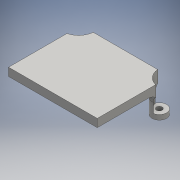
# Autodesk Inventor part: Fan bracket
Saved by Autodesk Inventor 2016 (Build 200138000, 138)
## iProperties
Created: 2019-09-20
Part Number: Fan bracket
Material: Generic
Document SubType Name: Modeling
Designer: jimmy
Density: 1 g/cm^3
Appearance: Default
Author: jimmy
Autodesk Inventor part; units mm, degrees
ref_plane "YZ Plane" through (0, 0, 0) normal (1, 0, 0) x (0, 1, 0)
ref_plane "XZ Plane" through (0, 0, 0) normal (0, 1, 0) x (-1, 0, 0)
ref_plane "XY Plane" through (0, 0, 0) normal (0, 0, 1) x (1, 0, 0)
sketch "Sketch1" plane through (0, 0, 0) normal (0, 0, 1) x (1, 0, 0)
  line L0 (-27.5, 22.5) -> (27.5, 22.5)
  line L1 (27.5, 22.5) -> (27.5, -22.5)
  line L2 (27.5, -22.5) -> (-27.5, -22.5)
  line L3 (-27.5, -22.5) -> (-27.5, 22.5)
  line L4 (-27.5, 22.5) -> (27.5, -22.5) construction
  line L5 (27.5, 22.5) -> (-27.5, -22.5) construction
  point P0 (0, 0)
  dimension "d0" = 55
  dimension "d1" = 45
  constraints: 12 end point, 2 midpoint, 2 parallel, 1 horizontal, 1 perpendicular
  measures "d0" distance of L1.end L2.end
  measures "d1" distance of L0.end L1.end
extrude "Extrusion1" add sketch "Sketch1" along normal blind 5
sketch "Sketch2" plane through (0, 0, 5) normal (0, 0, 1) x (1, 0, 0)
  line L0 (27.5, 22.5) -> (-27.5, 22.5) projected
  line L1 (-27.5, 22.5) -> (-27.5, -22.5) projected
  line L2 (-27.5, -22.5) -> (27.5, -22.5) projected
  line L3 (27.5, -22.5) -> (27.5, 22.5) projected
  line L4 (27.5, 22.5) -> (-27.5, 22.5) projected
  line L5 (27.5, -22.5) -> (27.5, 22.5) projected
  line L6 (-27.5, 22.5) -> (-27.5, -22.5) projected
  circle A0 centre (-24.5, 19) radius 4.5
  circle A1 centre (24.5, 19) radius 4.5
  line L7 (-40.6, 0) -> (40.6, 0) construction
  line L8 (0, -31.5) -> (0, 31.5) construction
  line L9 (-24.5, 19) -> (24.5, 19)
  point P0 (0, 0)
  point P1 (0, 19)
  dimension "d19" = 9
  dimension "d20" = 9
  dimension "d30" = 49
  dimension "d31" = 3.5
  constraints: 2 centre point, 2 end point, 1 horizontal, 1 midpoint, 1 point on line
  measures "d19" diameter of A0
  measures "d20" diameter of A1
  measures "d30" distance of L9.start L9.end
  measures "d31" distance between parallel lines of L9 L0
extrude "Extrusion2" add sketch "Sketch2" against normal blind 20 contours A1 L3 L0 | L0 A1 | A1 L3 | A0 L1 L0 | L0 A0 | L1 A0 picked at (23.9815, 19.6233) picked at (-23.4271, 18.4067)
sketch "Sketch3" plane through (0, 0, 5) normal (0, 0, 1) x (1, 0, 0)
  line L0 (-27.5, 22.5) -> (-27.3284, 22.5) projected
  line L1 (27.5, 22.5) -> (27.5, 22.3541) projected
  line L2 (27.5, -22.5) -> (-27.5, -22.5) projected
  line L3 (-27.5, -22.5) -> (-27.5, 15.6459) projected
  circle A0 centre (-24.5, 19) radius 3
  line L4 (-16.6703, 13.7531) -> (-27.5, 13.7531) construction
  line L5 (-20, 11.9289) -> (-20, 22.5) construction
  arc A1 (-27.5, 13.7531) -> (-20, 22.5) centre (-29.7996, 23.3138) ccw
  line L6 (21.6716, 22.5) -> (-21.6716, 22.5) projected
  line L7 (-27.5, 15.6459) -> (-27.5, -22.5) projected
  arc A2 (21.6716, 22.5) -> (27.5, 15.6459) centre (24.5, 19) ccw projected
  arc A3 (-27.5, 15.6459) -> (-21.6716, 22.5) centre (-24.5, 19) ccw projected
  line L8 (-20, 22.5) -> (-20, 25.8923)
  line L9 (-20, 25.8923) -> (-33.1535, 25.8923)
  line L10 (-33.1535, 25.8923) -> (-33.1535, 13.7531)
  line L11 (-33.1535, 13.7531) -> (-27.5, 13.7531)
  arc A4 (27.5, 22.3541) -> (27.3284, 22.5) centre (24.5, 19) ccw projected
  line L12 (27.3284, 22.5) -> (27.5, 22.5) projected
  line L13 (27.5, 15.6459) -> (27.5, -22.5) projected
  line L14 (-21.6716, 22.5) -> (21.6716, 22.5) projected
  arc A5 (-27.3284, 22.5) -> (-27.5, 22.3541) centre (-24.5, 19) ccw projected
  line L15 (-27.5, 22.3541) -> (-27.5, 22.5) projected
  point P0 (0, 0)
  point P1 (-22.5, 17.5)
  point P2 (22.5, 17.5)
  dimension "d11" = 6
  constraints: 12 end point, 3 perpendicular, 2 centre point, 2 point on circle, 2 tangent, 2 vertical, 1 coincident, 1 collinear, 1 point on line, 2 other
  measures "d11" diameter of A0
extrude "Extrusion4" cut sketch "Sketch3" against normal blind 17 contours L0 A5 L15 | A0 | L11 L10 L9 L8 L6 A3 A1 L3 | L3 A3 A1 | A1 A3 L6
sketch "Sketch5" plane through (0, 0, -12) normal (0, 0, 1) x (1, 0, 0)
  arc A0 (-20.3255, 20.6803) -> (-25.298, 14.5713) centre (-24.5, 19) ccw projected
  arc A1 (-25.298, 14.5713) -> (-20.3255, 20.6803) centre (-29.7996, 23.3138) ccw projected
  circle A2 centre (-24.5, 19) radius 1.75
  point P0 (0, 0)
  dimension "d27" = 3.5
  constraints: 1 centre point, 1 coincident
  measures "d27" diameter of A2
extrude "Extrusion5" cut sketch "Sketch5" against normal blind 17 contours A2
mirror "Mirror2" about plane through (0, 0, 0) normal (1, 0, 0) of "Extrusion4", "Extrusion5"
fillet "Fillet1" radius 6 2 edges at (-20.0821, 19.8558, 0) (-21.6139, 15.5474, 0)
mirror "Mirror3" about plane through (0, 0, 0) normal (1, 0, 0) of "Fillet1"
equation "\"d20\" = d19"
body "Solid1"
